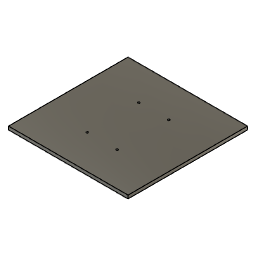
Pracovni deska v1 (Autodesk Fusion 360 design; units mm, degrees)
Autodesk Fusion 360 part; units mm, degrees
sketch "Sketch1" plane through (0, 0, 0) normal (0, 0, 1) x (1, 0, 0)
  line L0 (0, 0) -> (220, 0)
  line L1 (220, 0) -> (220, 220)
  line L2 (220, 220) -> (0, 220)
  line L3 (0, 220) -> (0, 0)
  circle A0 centre (82.5, 62.5) radius 1.75
  circle A1 centre (137.5, 62.5) radius 1.75
  circle A2 centre (82.5, 157.5) radius 1.75
  circle A3 centre (137.5, 157.5) radius 1.75
  dimension "d3" = 220
  dimension "d5" = 3.5
  dimension "d6" = 82.5
  dimension "d9" = 220
  dimension "d10" = 220
  dimension "d11" = 220
  dimension "d13" = 62.5
  dimension "d16" = 55
  dimension "d17" = 95
  dimension "d18" = 95
  dimension "d19" = 82.5
  constraint horizontal L0
  constraint vertical L1
  constraint horizontal L2
  constraint vertical L3
  measures "d3" distance of L1.end L2.end
  measures "d5" diameter of A0
  measures "d6" horizontal distance of L0.start A0.centre
  measures "d9" distance of L0.start L0.end
  measures "d10" distance of L0.start L2.end
  measures "d11" distance of L0.end L1.end
  measures "d13" vertical distance of L0.start A0.centre
  measures "d19" horizontal distance of L1.end A3.centre
extrude "Extrude1" add sketch "Sketch1" along normal blind 6
